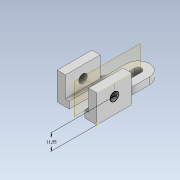
# Autodesk Inventor part: BeltDiscBottomPar_ohneLagert
Saved by Autodesk Inventor 2022 (Build 260153000, 153)
## iProperties
Created: 2022-10-05
Part Number: BeltDiscBottomPar_ohneLagert
Material: Generisch
Document SubType Name: Modeling
Designer: alexw
Density: 1 g/cm^3
Appearance: Vorgabe
Author: alexw
Autodesk Inventor part; units mm, degrees
ref_plane "YZ Plane" through (0, 0, 0) normal (1, 0, 0) x (0, 1, 0)
ref_plane "XZ Plane" through (0, 0, 0) normal (0, 1, 0) x (-1, 0, 0)
ref_plane "XY Plane" through (0, 0, 0) normal (0, 0, 1) x (1, 0, 0)
sketch "Skizze1" plane through (0, 0, 0) normal (0, 0, 1) x (1, 0, 0)
  line L0 (0, 0) -> (0, 20)
  line L1 (0, 20) -> (6, 20)
  line L2 (6, 20) -> (6, 5)
  line L3 (6, 5) -> (22.5, 5)
  line L4 (22.5, 5) -> (22.5, 20)
  line L5 (22.5, 20) -> (28.5, 20)
  line L6 (28.5, 20) -> (28.5, 0)
  line L7 (28.5, 0) -> (0, 0)
  line L8 (14.25, 5) -> (14.25, 0) construction
  line L9 (0, 11.55) -> (28.5, 11.55) construction
  dimension "d0" = 6
  dimension "d1" = 5
  dimension "d2" = 11.55
  dimension "d3" = 16.5
  dimension "d4" = 20
  dimension "d14" = 28.5
  constraints: 20 end point, 6 perpendicular, 4 point on line, 2 midpoint, 2 vertical, 1 collinear, 1 horizontal
  measures "d0" distance between parallel lines of L0 L2
  measures "d1" distance between parallel lines of L3 L7
  measures "d2" distance between parallel lines of L9 L7
  measures "d3" distance between parallel lines of L4 L2
  measures "d4" distance of L0.start L0.end
  measures "d14" distance between parallel lines of L6 L0
extrude "Extrusion1" add sketch "Skizze1" along normal blind 25
sketch "Skizze2" plane through (28.5, 0, 0) normal (1, 0, 0) x (0, 0, -1)
  line L0 (-12.5, 11.55) -> (-12.5, 20) construction
  line L1 (0, 20) -> (-25, 20) construction
  circle A0 centre (-12.5, 11.55) radius 3
  point P0 (0, 0)
  point P1 (-25, 0)
  dimension "d7" = 11.55
  dimension "d20" = 6
  constraints: 2 end point, 1 centre point, 1 coincident, 1 midpoint, 1 vertical
  measures "d7" vertical distance of L0.start point (-25, 0)
  measures "d20" diameter of A0
extrude "Extrusion2" cut sketch "Skizze2" against normal through all
sketch "Skizze3" plane through (6, 5, 0) normal (0, 1, 0) x (1, 0, 0)
  line L0 (16.5, -25) -> (0, -25) construction
  line L1 (8.25, -25) -> (8.25, 0) construction
  line L2 (16.5, 0) -> (0, 0) construction
  line L3 (8.25, -43.5) -> (8.25, -6.5) construction
  line L4 (13.75, -43.5) -> (13.75, -6.5)
  line L5 (2.75, -6.5) -> (2.75, -43.5)
  arc A0 (2.75, -43.5) -> (13.75, -43.5) centre (8.25, -43.5) ccw
  arc A1 (13.75, -6.5) -> (2.75, -6.5) centre (8.25, -6.5) ccw
  line L6 (28.2, -12.5) -> (-11.7, -12.5) construction
  point P0 (-6, 0)
  dimension "d11" = 11
  dimension "d25" = 6
  constraints: 10 end point, 4 point on circle, 4 tangent, 3 midpoint, 2 centre point, 1 parallel, 1 point on line
  measures "d11" distance between parallel lines of L4 L5
  measures "d25" distance from line of L3.end L6
extrude "Extrusion3" cut sketch "Skizze3" against normal through all
sketch "Skizze4" plane through (6, 5, 0) normal (0, 1, 0) x (1, 0, 0)
  line L0 (16.5, 0) -> (0, 0) projected
  line L1 (8.25, -11) -> (8.25, 19) construction
  line L2 (-6, 0) -> (22.5, 0) projected
  line L3 (0, -11) -> (0, 19)
  line L4 (16.5, 19) -> (16.5, -11)
  arc A0 (0, -11) -> (16.5, -11) centre (8.25, -11) ccw
  arc A1 (16.5, 19) -> (0, 19) centre (8.25, 19) ccw
  line L5 (5.75, 19) -> (5.75, -11)
  arc A2 (5.75, -11) -> (10.75, -11) centre (8.25, -11) ccw
  line L6 (10.75, -11) -> (10.75, 19)
  arc A3 (10.75, 19) -> (5.75, 19) centre (8.25, 19) ccw
  arc A4 (5.75, 6.5) -> (10.75, 6.5) centre (8.25, 6.5) ccw
  point P0 (8.25, 4)
  point P1 (16.5, 0)
  point P2 (5.75, 0)
  point P3 (10.75, 0)
  point P4 (8.25, 0)
  point P5 (8.25, 0)
  dimension "d15" = 15
  dimension "d18" = 5
  dimension "d26" = 4
  constraints: 12 end point, 11 point on circle, 6 tangent, 5 centre point, 4 point on line, 2 midpoint, 2 parallel, 1 perpendicular, 3 other
  measures "d15" distance of point (8.25, 4) L1.end
  measures "d18" distance between parallel lines of L6 L5
  measures "d26" distance from line of point (8.25, 4) L0
extrude "Extrusion4" add sketch "Skizze4" against normal up to surface (5 mm away) contours L0 L6 A3 L5 L3 A1 L4 | L0 L5 A4 L6
fillet "Rundung1" radius 6 2 edges at (6, 2.5, 0) (22.5, 2.5, 0)
ref_plane "Arbeitsebene1" through (14.25, 0, 25) normal (1, 0, 0) x (0, 0, -1)
